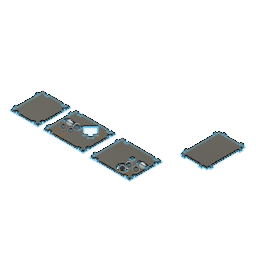
BoxForPunchy (Autodesk Fusion 360 design; units mm, degrees)
Autodesk Fusion 360 part; units mm, degrees
sketch "Sketch1" plane through (0, 0, 0) normal (0, 0, 1) x (1, 0, 0)
  line L0 (397.6682, 205.6704) -> (397.6682, 211.6704)
  line L1 (397.6682, 211.6704) -> (387.6682, 211.6704)
  line L2 (387.6682, 211.6704) -> (387.6682, 205.6704)
  line L3 (467.6682, 205.6704) -> (467.6682, 211.6704)
  line L4 (467.6682, 211.6704) -> (457.6682, 211.6704)
  line L5 (457.6682, 211.6704) -> (457.6682, 205.6704)
  line L6 (381.6682, 45.6704) -> (391.6682, 45.6704)
  line L7 (391.6682, 45.6704) -> (391.6682, 51.6704)
  line L8 (381.6682, 51.6704) -> (381.6682, 45.6704)
  line L9 (451.6682, 45.6704) -> (461.6682, 45.6704)
  line L10 (461.6682, 45.6704) -> (461.6682, 51.6704)
  line L11 (451.6682, 51.6704) -> (451.6682, 45.6704)
  line L12 (476.6682, 190.6704) -> (482.6682, 190.6704)
  line L13 (482.6682, 190.6704) -> (482.6682, 180.6704)
  line L14 (482.6682, 180.6704) -> (476.6682, 180.6704)
  line L15 (476.6682, 70.6704) -> (482.6682, 70.6704)
  line L16 (482.6682, 70.6704) -> (482.6682, 60.6704)
  line L17 (482.6682, 60.6704) -> (476.6682, 60.6704)
  line L18 (366.6682, 196.6704) -> (372.6682, 196.6704)
  line L19 (372.6682, 186.6704) -> (366.6682, 186.6704)
  line L20 (366.6682, 186.6704) -> (366.6682, 196.6704)
  line L21 (366.6682, 76.6704) -> (372.6682, 76.6704)
  line L22 (372.6682, 66.6704) -> (366.6682, 66.6704)
  line L23 (366.6682, 66.6704) -> (366.6682, 76.6704)
  line L24 (387.6682, 205.6704) -> (372.6682, 205.6704)
  line L25 (372.6682, 205.6704) -> (372.6682, 196.6704)
  line L26 (372.6682, 186.6704) -> (372.6682, 76.6704)
  line L27 (372.6682, 66.6704) -> (372.6682, 51.6704)
  line L28 (372.6682, 51.6704) -> (381.6682, 51.6704)
  line L29 (391.6682, 51.6704) -> (451.6682, 51.6704)
  line L30 (461.6682, 51.6704) -> (476.6682, 51.6704)
  line L31 (476.6682, 51.6704) -> (476.6682, 60.6704)
  line L32 (476.6682, 70.6704) -> (476.6682, 180.6704)
  line L33 (476.6682, 190.6704) -> (476.6682, 205.6704)
  line L34 (476.6682, 205.6704) -> (467.6682, 205.6704)
  line L35 (457.6682, 205.6704) -> (397.6682, 205.6704)
  line L36 (-132.3216, -142.5341) -> (-117.3216, -142.5341)
  line L37 (-138.3216, -37.5341) -> (-132.3216, -37.5341)
  line L38 (-138.3216, -127.5341) -> (-138.3216, -117.5341)
  line L39 (-47.3216, -12.5341) -> (-107.3216, -12.5341)
  line L40 (-37.3216, -12.5341) -> (-37.3216, -18.5341)
  line L41 (-47.3216, -18.5341) -> (-47.3216, -12.5341)
  line L42 (-107.3216, -18.5341) -> (-117.3216, -18.5341)
  line L43 (-22.3216, -142.5341) -> (-22.3216, -127.5341)
  line L44 (-117.3216, -12.5341) -> (-132.3216, -12.5341)
  line L45 (-22.3216, -117.5341) -> (-22.3216, -37.5341)
  line L46 (-132.3216, -12.5341) -> (-132.3216, -27.5341)
  line L47 (-37.3216, -142.5341) -> (-22.3216, -142.5341)
  line L48 (-28.3216, -37.5341) -> (-28.3216, -27.5341)
  line L49 (-117.3216, -18.5341) -> (-117.3216, -12.5341)
  line L50 (-28.3216, -117.5341) -> (-22.3216, -117.5341)
  line L51 (-132.3216, -27.5341) -> (-138.3216, -27.5341)
  line L52 (-22.3216, -27.5341) -> (-22.3216, -12.5341)
  line L53 (-107.3216, -12.5341) -> (-107.3216, -18.5341)
  line L54 (-132.3216, -37.5341) -> (-132.3216, -117.5341)
  line L55 (-37.3216, -136.5341) -> (-47.3216, -136.5341)
  line L56 (-107.3216, -136.5341) -> (-117.3216, -136.5341)
  line L57 (-37.3216, -18.5341) -> (-47.3216, -18.5341)
  line L58 (-22.3216, -37.5341) -> (-28.3216, -37.5341)
  line L59 (-132.3216, -127.5341) -> (-132.3216, -142.5341)
  line L60 (-138.3216, -27.5341) -> (-138.3216, -37.5341)
  line L61 (-47.3216, -136.5341) -> (-47.3216, -142.5341)
  line L62 (-28.3216, -27.5341) -> (-22.3216, -27.5341)
  line L63 (-117.3216, -136.5341) -> (-117.3216, -142.5341)
  line L64 (-132.3216, -127.5341) -> (-138.3216, -127.5341)
  line L65 (-107.3216, -142.5341) -> (-107.3216, -136.5341)
  line L66 (-28.3216, -127.5341) -> (-28.3216, -117.5341)
  line L67 (-22.3216, -12.5341) -> (-37.3216, -12.5341)
  line L68 (-22.3216, -127.5341) -> (-28.3216, -127.5341)
  line L69 (-138.3216, -117.5341) -> (-132.3216, -117.5341)
  line L70 (-37.3216, -142.5341) -> (-37.3216, -136.5341)
  line L71 (-107.3216, -142.5341) -> (-47.3216, -142.5341)
  line L72 (192.1859, -41.4802) -> (198.1859, -41.4802)
  line L73 (4.4052, -128.4307) -> (-1.5948, -128.4307)
  line L74 (198.1859, -31.4802) -> (192.1859, -31.4802)
  line L75 (139.4052, -137.4307) -> (139.4052, -143.4307)
  line L76 (223.1859, -16.4802) -> (223.1859, -22.4802)
  line L77 (149.4052, -143.4307) -> (149.4052, -137.4307)
  line L78 (213.1859, -16.4802) -> (198.1859, -16.4802)
  line L79 (19.4052, -137.4307) -> (19.4052, -143.4307)
  line L80 (4.4052, -28.4307) -> (-1.5948, -28.4307)
  line L81 (149.4052, -13.4307) -> (149.4052, -19.4307)
  line L82 (29.4052, -137.4307) -> (19.4052, -137.4307)
  line L83 (158.4052, -118.4307) -> (164.4052, -118.4307)
  line L84 (139.4052, -13.4307) -> (29.4052, -13.4307)
  line L85 (198.1859, -41.4802) -> (198.1859, -121.4802)
  line L86 (343.1859, -146.4802) -> (358.1859, -146.4802)
  line L87 (352.1859, -121.4802) -> (358.1859, -121.4802)
  line L88 (343.1859, -140.4802) -> (333.1859, -140.4802)
  line L89 (358.1859, -16.4802) -> (343.1859, -16.4802)
  line L90 (343.1859, -146.4802) -> (343.1859, -140.4802)
  line L91 (333.1859, -140.4802) -> (333.1859, -146.4802)
  line L92 (352.1859, -31.4802) -> (358.1859, -31.4802)
  line L93 (198.1859, -131.4802) -> (192.1859, -131.4802)
  line L94 (198.1859, -16.4802) -> (198.1859, -31.4802)
  line L95 (19.4052, -13.4307) -> (4.4052, -13.4307)
  line L96 (213.1859, -140.4802) -> (213.1859, -146.4802)
  line L97 (-1.5948, -28.4307) -> (-1.5948, -38.4307)
  line L98 (4.4052, -143.4307) -> (19.4052, -143.4307)
  line L99 (164.4052, -13.4307) -> (149.4052, -13.4307)
  line L100 (4.4052, -38.4307) -> (4.4052, -118.4307)
  line L101 (19.4052, -19.4307) -> (19.4052, -13.4307)
  line L102 (164.4052, -38.4307) -> (158.4052, -38.4307)
  line L103 (-1.5948, -128.4307) -> (-1.5948, -118.4307)
  line L104 (223.1859, -140.4802) -> (213.1859, -140.4802)
  line L105 (29.4052, -143.4307) -> (29.4052, -137.4307)
  line L106 (158.4052, -28.4307) -> (164.4052, -28.4307)
  line L107 (-1.5948, -118.4307) -> (4.4052, -118.4307)
  line L108 (149.4052, -19.4307) -> (139.4052, -19.4307)
  line L109 (-1.5948, -38.4307) -> (4.4052, -38.4307)
  line L110 (358.1859, -41.4802) -> (352.1859, -41.4802)
  line L111 (343.1859, -16.4802) -> (343.1859, -22.4802)
  line L112 (4.4052, -128.4307) -> (4.4052, -143.4307)
  line L113 (192.1859, -121.4802) -> (198.1859, -121.4802)
  line L114 (29.4052, -13.4307) -> (29.4052, -19.4307)
  line L115 (139.4052, -19.4307) -> (139.4052, -13.4307)
  line L116 (4.4052, -13.4307) -> (4.4052, -28.4307)
  line L117 (192.1859, -31.4802) -> (192.1859, -41.4802)
  line L118 (358.1859, -121.4802) -> (358.1859, -41.4802)
  line L119 (192.1859, -131.4802) -> (192.1859, -121.4802)
  line L120 (223.1859, -146.4802) -> (333.1859, -146.4802)
  line L121 (164.4052, -118.4307) -> (164.4052, -38.4307)
  line L122 (223.1859, -22.4802) -> (213.1859, -22.4802)
  line L123 (164.4052, -28.4307) -> (164.4052, -13.4307)
  line L124 (29.4052, -19.4307) -> (19.4052, -19.4307)
  line L125 (343.1859, -22.4802) -> (333.1859, -22.4802)
  line L126 (352.1859, -131.4802) -> (352.1859, -121.4802)
  line L127 (29.4052, -143.4307) -> (139.4052, -143.4307)
  line L128 (358.1859, -31.4802) -> (358.1859, -16.4802)
  line L129 (333.1859, -22.4802) -> (333.1859, -16.4802)
  line L130 (158.4052, -38.4307) -> (158.4052, -28.4307)
  line L131 (158.4052, -128.4307) -> (158.4052, -118.4307)
  line L132 (333.1859, -16.4802) -> (223.1859, -16.4802)
  line L133 (164.4052, -128.4307) -> (158.4052, -128.4307)
  line L134 (213.1859, -22.4802) -> (213.1859, -16.4802)
  line L135 (358.1859, -131.4802) -> (352.1859, -131.4802)
  line L136 (358.1859, -146.4802) -> (358.1859, -131.4802)
  line L137 (352.1859, -41.4802) -> (352.1859, -31.4802)
  line L138 (149.4052, -143.4307) -> (164.4052, -143.4307)
  line L139 (198.1859, -131.4802) -> (198.1859, -146.4802)
  line L140 (198.1859, -146.4802) -> (213.1859, -146.4802)
  line L141 (164.4052, -143.4307) -> (164.4052, -128.4307)
  line L142 (223.1859, -146.4802) -> (223.1859, -140.4802)
  line L143 (149.4052, -137.4307) -> (139.4052, -137.4307)
  line L144 (302.1859, -146.4802) -> (302.1859, -120.4802) construction
  circle A0 centre (302.1859, -120.4802) radius 17.5
  line L145 (302.1859, -146.4802) -> (302.1859, -93.8802) construction
  circle A1 centre (302.1859, -93.8802) radius 2.5
  line L146 (60.4052, -143.4307) -> (60.4052, -90.8307) construction
  circle A2 centre (60.4052, -90.8307) radius 2.5
  line L147 (332.1859, -146.4802) -> (332.1859, -94.4802) construction
  circle A3 centre (332.1859, -94.4802) radius 2.05
  circle A4 centre (30.4052, -91.4307) radius 2.05
  line L148 (30.4052, -143.4307) -> (30.4052, -91.4307) construction
  line L149 (74.1285, -52.7836) -> (104.0391, -22.8729)
  line L150 (104.0391, -22.8729) -> (133.9497, -52.7836)
  line L151 (104.0391, -82.6942) -> (74.1285, -52.7836)
  line L152 (124.6513, -62.082) -> (133.8436, -71.2744)
  line L153 (133.8436, -71.2744) -> (122.5299, -82.5881)
  line L154 (122.5299, -82.5881) -> (113.3375, -73.3957)
  line L155 (164.4052, -54.4307) -> (134.4052, -54.4307) construction
  line L156 (134.4052, -19.4307) -> (134.4052, -54.4307) construction
  line L157 (332.1859, -94.4802) -> (358.1859, -94.4802) construction
  line L158 (30.4052, -91.4307) -> (4.4052, -91.4307) construction
  line L159 (30.4052, -65.6935) -> (60.4052, -65.6935) construction
  line L160 (30.4052, -91.4307) -> (30.4052, -65.4307) construction
  circle A5 centre (60.4052, -65.6935) radius 2.5
  line L161 (133.9497, -52.7836) -> (124.6513, -62.082)
  line L162 (113.3375, -73.3957) -> (104.0391, -82.6942)
  line L163 (30.4052, -133.2522) -> (60.4052, -133.2522) construction
  line L164 (302.1859, -133.9917) -> (332.1859, -133.9917) construction
  line L165 (13.6269, -70.0961) -> (48.6269, -70.0961)
  line L166 (48.6269, -70.0961) -> (48.6269, -60.0961)
  line L167 (48.6269, -60.0961) -> (13.6269, -60.0961)
  line L168 (13.6269, -60.0961) -> (13.6269, -70.0961)
  line L169 (66.4175, -60.1949) -> (76.4175, -60.1949)
  line L170 (76.4175, -60.1949) -> (76.4175, -70.1949)
  line L171 (76.4175, -70.1949) -> (66.4175, -70.1949)
  line L172 (66.4175, -70.1949) -> (66.4175, -60.1949)
  line L173 (332.1859, -94.4802) -> (332.1859, -68.4802) construction
  line L174 (314.7934, -62.0421) -> (349.7934, -62.0421)
  line L175 (349.7934, -62.0421) -> (349.7934, -72.0421)
  line L176 (349.7934, -72.0421) -> (314.7934, -72.0421)
  line L177 (314.7934, -72.0421) -> (314.7934, -62.0421)
  line L178 (284.9855, -62.3266) -> (294.9855, -62.3266)
  line L179 (294.9855, -62.3266) -> (294.9855, -72.3266)
  line L180 (294.9855, -72.3266) -> (284.9855, -72.3266)
  line L181 (284.9855, -72.3266) -> (284.9855, -62.3266)
  dimension "d125" = 104
  dimension "d126" = 154
  dimension "d127" = 10
  dimension "d129" = 10
  dimension "d130" = 6
  dimension "d131" = 10
  dimension "d133" = 10
  dimension "d134" = 6
  dimension "d135" = 6
  dimension "d136" = 10
  dimension "d137" = 6
  dimension "d138" = 10
  dimension "d139" = 6
  dimension "d140" = 10
  dimension "d141" = 6
  dimension "d142" = 10
  dimension "d151" = 110
  dimension "d152" = 130
  dimension "d153" = 10
  dimension "d154" = 6
  dimension "d155" = 15
  dimension "d156" = 10
  dimension "d157" = 6
  dimension "d158" = 15
  dimension "d159" = 10
  dimension "d160" = 6
  dimension "d161" = 10
  dimension "d162" = 6
  dimension "d163" = 15
  dimension "d164" = 15
  dimension "d165" = 6
  dimension "d166" = 10
  dimension "d167" = 6
  dimension "d168" = 10
  dimension "d169" = 6
  dimension "d170" = 10
  dimension "d171" = 6
  dimension "d172" = 10
  dimension "d173" = 15
  dimension "d174" = 15
  dimension "d175" = 15
  dimension "d176" = 15
  dimension "d177" = 160
  dimension "d178" = 130
  dimension "d179" = 10
  dimension "d180" = 6
  dimension "d181" = 15
  dimension "d182" = 10
  dimension "d183" = 6
  dimension "d184" = 15
  dimension "d185" = 10
  dimension "d186" = 6
  dimension "d187" = 10
  dimension "d188" = 6
  dimension "d189" = 15
  dimension "d190" = 15
  dimension "d191" = 6
  dimension "d192" = 10
  dimension "d193" = 6
  dimension "d194" = 10
  dimension "d195" = 6
  dimension "d196" = 10
  dimension "d197" = 6
  dimension "d198" = 10
  dimension "d199" = 15
  dimension "d200" = 15
  dimension "d201" = 15
  dimension "d202" = 15
  dimension "d203" = 160
  dimension "d204" = 130
  dimension "d205" = 10
  dimension "d206" = 6
  dimension "d207" = 15
  dimension "d208" = 10
  dimension "d209" = 6
  dimension "d210" = 15
  dimension "d211" = 10
  dimension "d212" = 6
  dimension "d213" = 10
  dimension "d214" = 6
  dimension "d215" = 15
  dimension "d216" = 15
  dimension "d217" = 6
  dimension "d218" = 10
  dimension "d219" = 6
  dimension "d220" = 10
  dimension "d221" = 6
  dimension "d222" = 10
  dimension "d223" = 6
  dimension "d224" = 10
  dimension "d225" = 15
  dimension "d226" = 15
  dimension "d227" = 15
  dimension "d228" = 15
  dimension "d229" = 26
  dimension "d230" = 35
  dimension "d233" = 60
  dimension "d234" = 110
  dimension "d235" = 60
  dimension "d236" = 110
  dimension "d237" = 6
  dimension "d238" = 15
  dimension "d239" = 15
  dimension "d240" = 15
  dimension "d241" = 15
  dimension "d244" = 6
  dimension "d245" = 52.6
  dimension "d246" = 5
  dimension "d247" = 52.6
  dimension "d248" = 5
  dimension "d249" = 52
  dimension "d251" = 4.1
  dimension "d252" = 52
  dimension "d254" = 4.1
  dimension "d265" = 42.3
  dimension "d266" = 42.3
  dimension "d267" = 16
  dimension "d268" = 13
  dimension "d269" = 30
  dimension "d270" = 35
  dimension "d271" = 26
  dimension "d272" = 26
  dimension "d273" = 30
  dimension "d274" = 26
  dimension "d275" = 5
  dimension "d282" = 30
  dimension "d283" = 30
  dimension "d284" = 35
  dimension "d285" = 10
  dimension "d286" = 10
  dimension "d287" = 10
  dimension "d288" = 26
  dimension "d289" = 35
  dimension "d290" = 10
  dimension "d291" = 10
  dimension "d292" = 10
  constraint horizontal L28
  constraint vertical L31
  constraint horizontal L34
  constraint vertical L25
  constraint vertical L0
  constraint horizontal L1
  constraint vertical L2
  constraint vertical L3
  constraint horizontal L4
  constraint vertical L5
  constraint horizontal L6
  constraint vertical L7
  constraint vertical L8
  constraint horizontal L9
  constraint vertical L10
  constraint vertical L11
  constraint horizontal L12
  constraint vertical L13
  constraint horizontal L14
  constraint horizontal L15
  constraint vertical L16
  constraint horizontal L17
  constraint horizontal L18
  constraint horizontal L19
  constraint vertical L20
  constraint horizontal L21
  constraint horizontal L22
  constraint vertical L23
  constraint coincident L2.end L34
  constraint coincident L5.end L34
  constraint coincident L12.start L31
  constraint coincident L15.start L31
  constraint coincident L21.end L25
  constraint coincident L10.end L28
  constraint coincident L7.end L28
  constraint collinear L24 L34
  constraint collinear L25 L26
  constraint collinear L26 L27
  constraint collinear L28 L29
  constraint collinear L29 L30
  constraint collinear L31 L32
  constraint collinear L32 L33
  constraint collinear L34 L35
  constraint horizontal L36
  constraint vertical L43
  constraint horizontal L67
  constraint vertical L46
  constraint vertical L53
  constraint horizontal L42
  constraint vertical L49
  constraint coincident L44.start L67
  constraint collinear L44 L67
  constraint vertical L40
  constraint horizontal L57
  constraint vertical L41
  constraint coincident L39.start L67
  constraint collinear L39 L67
  constraint vertical L65
  constraint horizontal L56
  constraint vertical L63
  constraint vertical L70
  constraint horizontal L55
  constraint vertical L61
  constraint coincident L47.start L36
  constraint collinear L36 L71
  constraint collinear L47 L71
  constraint horizontal L51
  constraint vertical L60
  constraint horizontal L37
  constraint horizontal L69
  constraint horizontal L64
  constraint vertical L38
  constraint horizontal L62
  constraint horizontal L58
  constraint vertical L48
  constraint horizontal L50
  constraint horizontal L68
  constraint vertical L66
  constraint coincident L54.end L46
  constraint coincident L52.start L43
  constraint coincident L45.start L43
  constraint collinear L46 L54
  constraint collinear L54 L59
  constraint collinear L43 L45
  constraint collinear L45 L52
  constraint horizontal L98
  constraint vertical L141
  constraint horizontal L99
  constraint vertical L116
  constraint vertical L114
  constraint horizontal L124
  constraint vertical L101
  constraint coincident L95.start L99
  constraint collinear L95 L99
  constraint vertical L81
  constraint horizontal L108
  constraint vertical L115
  constraint coincident L84.start L99
  constraint collinear L84 L99
  constraint vertical L105
  constraint horizontal L82
  constraint vertical L79
  constraint vertical L77
  constraint horizontal L143
  constraint vertical L75
  constraint coincident L77.start L98
  constraint collinear L98 L127
  constraint collinear L127 L138
  constraint horizontal L80
  constraint vertical L97
  constraint horizontal L109
  constraint horizontal L107
  constraint horizontal L73
  constraint vertical L103
  constraint horizontal L106
  constraint horizontal L102
  constraint vertical L130
  constraint horizontal L83
  constraint horizontal L133
  constraint vertical L131
  constraint coincident L100.end L116
  constraint coincident L106.end L141
  constraint coincident L83.end L141
  constraint collinear L100 L116
  constraint collinear L100 L112
  constraint collinear L121 L141
  constraint collinear L121 L123
  constraint horizontal L140
  constraint vertical L136
  constraint horizontal L89
  constraint vertical L94
  constraint vertical L76
  constraint horizontal L122
  constraint vertical L134
  constraint coincident L78.start L89
  constraint collinear L78 L89
  constraint vertical L111
  constraint horizontal L125
  constraint vertical L129
  constraint coincident L129.end L89
  constraint collinear L89 L132
  constraint vertical L142
  constraint horizontal L104
  constraint vertical L96
  constraint vertical L90
  constraint horizontal L88
  constraint vertical L91
  constraint coincident L86.start L140
  constraint collinear L120 L140
  constraint collinear L86 L120
  constraint horizontal L74
  constraint vertical L117
  constraint horizontal L72
  constraint horizontal L113
  constraint horizontal L93
  constraint vertical L119
  constraint horizontal L92
  constraint horizontal L110
  constraint vertical L137
  constraint horizontal L87
  constraint horizontal L135
  constraint vertical L126
  constraint coincident L85.end L94
  constraint coincident L92.end L136
  constraint coincident L87.end L136
  constraint collinear L85 L94
  constraint collinear L85 L139
  constraint collinear L118 L136
  constraint collinear L118 L128
  constraint perpendicular L120 L144
  constraint coincident L144.end A0.centre
  constraint perpendicular L120 L145
  constraint coincident L145.end A1.centre
  constraint perpendicular L127 L146
  constraint coincident L146.end A2.centre
  constraint coincident L120 L147.start
  constraint perpendicular L120 L147
  constraint coincident L147.end A3.centre
  constraint coincident A4.centre L148.end
  constraint vertical L148
  constraint coincident L127 L148.start
  constraint coincident L121 L155.start
  constraint perpendicular L121 L155
  constraint coincident L108 L156.start
  constraint perpendicular L108 L156
  constraint coincident L155.end L156.end
  constraint perpendicular L147 L157
  constraint coincident L118 L157.end
  constraint perpendicular L148 L158
  constraint coincident L100 L158.end
  constraint coincident L148 L159.start
  constraint perpendicular L148 L159
  constraint perpendicular L158 L160
  constraint coincident L159.end A5.centre
  constraint collinear L161 L162
  constraint coincident L127 L146.start
  constraint coincident L120 L144.start
  constraint coincident L148 L163.start
  constraint coincident L146 L163.end
  constraint perpendicular L146 L163
  constraint coincident L145 L164.start
  constraint coincident L147 L164.end
  constraint perpendicular L147 L164
  constraint horizontal L165
  constraint vertical L166
  constraint horizontal L167
  constraint vertical L168
  constraint horizontal L169
  constraint vertical L170
  constraint horizontal L171
  constraint vertical L172
  constraint perpendicular L157 L173
  constraint horizontal L174
  constraint vertical L175
  constraint horizontal L176
  constraint vertical L177
  constraint horizontal L178
  constraint vertical L179
  constraint horizontal L180
  constraint vertical L181
  measures "d125" distance of L27.end L30.end
  measures "d126" distance of L27.end L24.end
  measures "d127" distance of L2.end L0.start
  measures "d129" distance of L5.end L3.start
  measures "d130" distance of L5.end L4.end
  measures "d131" distance of L6.start L6.end
  measures "d133" distance of L9.start L9.end
  measures "d134" distance of L9.start L11.start
  measures "d135" distance of L12.start L12.end
  measures "d136" distance of L12.start L14.end
  measures "d137" distance of L15.start L15.end
  measures "d138" distance of L15.start L17.end
  measures "d139" distance of L18.start L18.end
  measures "d140" distance of L18.start L19.end
  measures "d141" distance of L21.start L21.end
  measures "d142" distance of L21.start L22.end
  measures "d151" distance of L36.start L43.start
  measures "d152" distance of L44.end L36.start
  measures "d153" distance of L39.end L44.start
  measures "d154" distance of L44.start L42.end
  measures "d155" distance of L44.end L44.start
  measures "d156" distance of L39.start L40.start
  measures "d157" distance of L39.start L41.start
  measures "d158" distance of L52.end L40.start
  measures "d159" distance of L36.end L65.start
  measures "d160" distance of L36.end L56.end
  measures "d161" distance of L47.start L61.end
  measures "d162" distance of L55.end L61.end
  measures "d163" distance of L47.start L43.start
  measures "d164" distance of L36.end L36.start
  measures "d165" distance of L46.end L51.end
  measures "d166" distance of L46.end L37.end
  measures "d167" distance of L38.end L54.end
  measures "d168" distance of L38.end L38.start
  measures "d169" distance of L48.end L52.start
  measures "d170" distance of L48.end L48.start
  measures "d171" distance of L50.start L45.start
  measures "d172" distance of L50.start L66.start
  measures "d173" distance of L46.end L44.end
  measures "d174" distance of L59.start L36.start
  measures "d175" distance of L52.end L52.start
  measures "d176" distance of L43.start L43.end
  measures "d177" distance of L98.start L138.end
  measures "d178" distance of L95.end L98.start
  measures "d179" distance of L84.end L95.start
  measures "d180" distance of L95.start L101.start
  measures "d181" distance of L95.end L95.start
  measures "d182" distance of L84.start L81.start
  measures "d183" distance of L84.start L108.end
  measures "d184" distance of L99.start L81.start
  measures "d185" distance of L79.end L105.start
  measures "d186" distance of L79.end L79.start
  measures "d187" distance of L77.start L75.end
  measures "d188" distance of L75.start L75.end
  measures "d189" distance of L77.start L138.end
  measures "d190" distance of L79.end L98.start
  measures "d191" distance of L80.start L80.end
  measures "d192" distance of L80.start L100.start
  measures "d193" distance of L103.end L100.end
  measures "d194" distance of L103.end L73.end
  measures "d195" distance of L106.start L106.end
  measures "d196" distance of L106.start L102.end
  measures "d197" distance of L83.start L83.end
  measures "d198" distance of L83.start L131.start
  measures "d199" distance of L80.start L95.end
  measures "d200" distance of L73.start L98.start
  measures "d201" distance of L99.start L106.end
  measures "d202" distance of L138.end L133.start
  measures "d203" distance of L139.end L86.end
  measures "d204" distance of L139.end L78.end
  measures "d205" distance of L78.start L76.start
  measures "d206" distance of L78.start L122.end
  measures "d207" distance of L78.start L78.end
  measures "d208" distance of L89.end L129.end
  measures "d209" distance of L129.end L125.end
  measures "d210" distance of L89.end L89.start
  measures "d211" distance of L120.start L96.end
  measures "d212" distance of L96.start L96.end
  measures "d213" distance of L91.end L86.start
  measures "d214" distance of L91.end L88.end
  measures "d215" distance of L86.start L86.end
  measures "d216" distance of L139.end L96.end
  measures "d217" distance of L74.end L74.start
  measures "d218" distance of L74.start L72.end
  measures "d219" distance of L113.start L85.end
  measures "d220" distance of L113.start L93.end
  measures "d221" distance of L92.start L92.end
  measures "d222" distance of L92.start L110.end
  measures "d223" distance of L87.end L87.start
  measures "d224" distance of L126.start L87.start
  measures "d225" distance of L74.start L78.end
  measures "d226" distance of L139.end L93.start
  measures "d227" distance of L92.end L89.start
  measures "d228" distance of L135.start L86.end
  measures "d229" distance of L144.start L144.end
  measures "d230" diameter of A0
  measures "d233" distance of L0.start L5.end
  measures "d234" distance of L14.end L15.start
  measures "d235" distance of L7.end L11.start
  measures "d236" distance of L19.start L21.end
  measures "d237" distance of L2.end L1.end
  measures "d238" distance of L27.end L22.start
  measures "d239" distance of L24.end L2.end
  measures "d240" distance of L33.end L12.start
  measures "d241" distance of L30.end L10.end
  measures "d244" distance of L6.end L7.end
  measures "d245" distance of L144.start L145.end
  measures "d246" diameter of A1
  measures "d247" distance of L146.start L146.end
  measures "d248" diameter of A2
  measures "d249" distance of L147.start L147.end
  measures "d251" diameter of A3
  measures "d252" distance of L148.start A4.centre
  measures "d254" diameter of A4
  measures "d265" distance of L149.start L149.end
  measures "d266" distance of L149.start L151.start
  measures "d267" distance of L154.end L152.start
  measures "d268" distance of L154.end L153.end
  measures "d269" distance of L155.start L155.end
  measures "d270" distance of L156.start L155.end
  measures "d271" distance of L147.end L157.end
  measures "d272" distance of A4.centre L158.end
  measures "d273" distance of L159.start L159.end
  measures "d274" distance of A4.centre L160.end
  measures "d275" diameter of A5
  measures "d282" distance of L163.start L163.end
  measures "d283" distance of L164.start L164.end
  measures "d284" distance of L165.start L165.end
  measures "d285" distance of L165.start L167.end
  measures "d286" distance of L169.start L169.end
  measures "d287" distance of L169.start L171.end
  measures "d288" distance of L147.end L173.end
  measures "d289" distance of L174.start L174.end
  measures "d290" distance of L174.start L176.end
  measures "d291" distance of L178.start L178.end
  measures "d292" distance of L178.start L180.end
extrude "Extrude3" add sketch "Sketch1" along normal blind 6 makes body 1 at (76.74, -126.6606, 0) makes body 2 at (227.1191, -78.429, 0) makes body 3 at (-80.9883, -64.2007, 0) makes body 4 at (407.3349, 148.0037, 0)
extrude "Extrude1" [suppressed]
copy_body "Body->Comp1" [suppressed] in component "Component"
equation "BoxWidth = 110 mm"
equation "BoxHeight = 130 mm"
equation "MaterialThickness = 6 mm"
equation "TabLength = 10 mm"
equation "d125 = BoxWidth - MaterialThickness"
equation "d126 = BoxLength - MaterialThickness"
equation "d127 = TabLength"
equation "d129 = TabLength"
equation "d130 = MaterialThickness"
equation "d131 = TabLength"
equation "d133 = TabLength"
equation "d134 = MaterialThickness"
equation "d135 = MaterialThickness"
equation "d136 = TabLength"
equation "d137 = MaterialThickness"
equation "d138 = TabLength"
equation "d139 = MaterialThickness"
equation "d140 = TabLength"
equation "d141 = MaterialThickness"
equation "d142 = TabLength"
equation "d153 = TabLength"
equation "d154 = MaterialThickness"
equation "d156 = TabLength"
equation "d157 = MaterialThickness"
equation "d159 = TabLength"
equation "d160 = MaterialThickness"
equation "d161 = TabLength"
equation "d162 = MaterialThickness"
equation "d165 = MaterialThickness"
equation "d166 = TabLength"
equation "d167 = MaterialThickness"
equation "d168 = TabLength"
equation "d169 = MaterialThickness"
equation "d170 = TabLength"
equation "d171 = MaterialThickness"
equation "d172 = TabLength"
equation "d177 = BoxLength"
equation "d179 = TabLength"
equation "d180 = MaterialThickness"
equation "d182 = TabLength"
equation "d183 = MaterialThickness"
equation "d185 = TabLength"
equation "d186 = MaterialThickness"
equation "d187 = TabLength"
equation "d188 = MaterialThickness"
equation "d191 = MaterialThickness"
equation "d192 = TabLength"
equation "d193 = MaterialThickness"
equation "d194 = TabLength"
equation "d195 = MaterialThickness"
equation "d196 = TabLength"
equation "d197 = MaterialThickness"
equation "d198 = TabLength"
equation "d203 = BoxLength"
equation "d205 = TabLength"
equation "d206 = MaterialThickness"
equation "d208 = TabLength"
equation "d209 = MaterialThickness"
equation "d211 = TabLength"
equation "d212 = MaterialThickness"
equation "d213 = TabLength"
equation "d214 = MaterialThickness"
equation "d217 = MaterialThickness"
equation "d218 = TabLength"
equation "d219 = MaterialThickness"
equation "d220 = TabLength"
equation "d221 = MaterialThickness"
equation "d222 = TabLength"
equation "d223 = MaterialThickness"
equation "d224 = TabLength"
equation "d229 = 20 mm + MaterialThickness"
equation "d237 = MaterialThickness"
equation "d244 = MaterialThickness"
equation "d245 = 48 mm + 4.6 mm"
equation "d247 = 48 mm + 4.6 mm"
equation "BoxLength = 160 mm"
